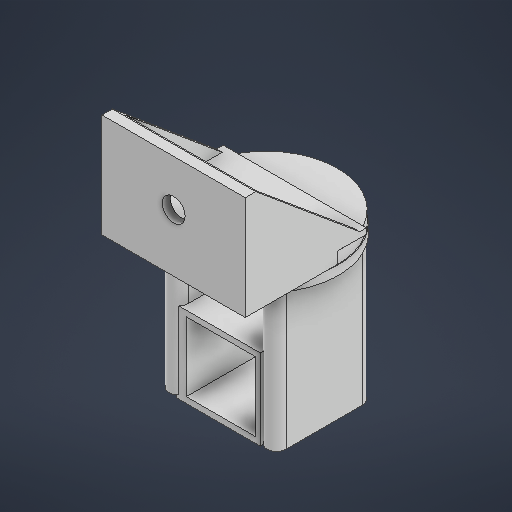
# Autodesk Inventor part: cam_mount0_WITHBASE
Saved by Autodesk Inventor 2027 (Build 310192060, 192F)
## iProperties
Created: 2026-07-16
Part Number: cam_mount0_WITHBASE
Material: Generic
Document SubType Name: Modeling
Designer: farde
Density: 1 g/cm^3
Appearance: Default
Author: farde
Autodesk Inventor part; units mm, degrees
ref_plane "YZ Plane" through (0, 0, 0) normal (1, 0, 0) x (0, 1, 0)
ref_plane "XZ Plane" through (0, 0, 0) normal (0, 1, 0) x (-1, 0, 0)
ref_plane "XY Plane" through (0, 0, 0) normal (0, 0, 1) x (1, 0, 0)
sketch "Sketch1" plane through (0, 0, 0) normal (0, 1, 0) x (-1, 0, 0)
  circle A0 centre (0, 0) radius 25.75
  circle A1 centre (0, 0) radius 23.5
  dimension "d0" = 51.5
  dimension "d1" = 47
  constraints: 2 centre point, 2 coincident
  measures "d0" diameter of A0
  measures "d1" diameter of A1
extrude "Extrusion1" add sketch "Sketch1" along normal blind 1
sketch "Sketch2" plane through (0, 0, 0) normal (0, 1, 0) x (-1, 0, 0)
  circle A0 centre (0, 0) radius 31.4135
  circle A1 centre (0, 0) radius 28.9404
  circle A2 centre (0, 0) radius 31.4135
  circle A3 centre (0, 0) radius 20.0919
  dimension "d6" = 40.1837
  constraints: 4 centre point, 4 coincident, 1 concentric
  measures "d6" diameter of A3
extrude "Extrusion2" add sketch "Sketch2" against normal blind 4 contours A0 | A1 | A3
sketch "Sketch3" plane through (0, -4, 0) normal (0, -1, 0) x (1, 0, 0)
  line L0 (21.2066, 16.5968) -> (21.2066, -16.5968) construction
  line L1 (17.0959, 16.5968) -> (17.0959, -16.5968)
  line L2 (25.3174, -16.5968) -> (25.3174, 16.5968)
  arc A0 (25.3174, 16.5968) -> (17.0959, 16.5968) centre (21.2066, 16.5968) ccw
  arc A1 (17.0959, -16.5968) -> (25.3174, -16.5968) centre (21.2066, -16.5968) ccw
  point P0 (0, 0)
  point P1 (21.2066, 0)
  dimension "d28" = 8.2215
  constraints: 8 end point, 4 point on circle, 4 tangent, 2 centre point, 1 midpoint, 1 parallel, 1 vertical
  measures "d28" distance between parallel lines of L1 L2
extrude "Extrusion3" add sketch "Sketch3" along normal blind 60
mirror "Mirror1" about plane through (0, 0, 0) normal (1, 0, 0) of "Extrusion3"
sketch "Sketch4" plane through (0, 0, 0) normal (0, 1, 0) x (1, 0, 0)
  circle A0 centre (0, 0) radius 17.5
  dimension "d11" = 35
  constraints: 1 centre point, 1 coincident
  measures "d11" diameter of A0
extrude "Extrusion4" cut sketch "Sketch4" against normal blind 60
sketch "Sketch5" plane through (17.0959, -64, -16.5968) normal (-1, 0, 0) x (0, 0, 1)
  line L0 (36.0968, -1.5251) -> (1.0968, -1.5251)
  line L1 (1.0968, -1.5251) -> (1.0968, 33.4749)
  line L2 (1.0968, 33.4749) -> (36.0968, 33.4749)
  line L3 (36.0968, 33.4749) -> (36.0968, -1.5251)
  line L4 (36.0968, -1.5251) -> (1.0968, 33.4749) construction
  line L5 (1.0968, -1.5251) -> (36.0968, 33.4749) construction
  point P0 (16.5968, 64)
  point P1 (18.5968, 15.9749)
  dimension "d12" = 35
  dimension "d13" = 35
  constraints: 12 end point, 2 midpoint, 2 parallel, 1 horizontal, 1 perpendicular
  measures "d12" distance of L1.end L2.end
  measures "d13" distance of L0.end L1.end
extrude "Extrusion5" add sketch "Sketch5" along normal blind 36.1875
sketch "Sketch6" plane through (17.0959, -65.5251, -15.5) normal (0, -1, 0) x (1, 0, 0)
  point P0 (-17.0959, 15.5)
sketch "Sketch8" plane through (-25.3174, -64, -16.5968) normal (-1, 0, 0) x (0, 0, 1)
  line L0 (11.7088, 49.275) -> (100.4099, 49.275) construction
  line L1 (100.4099, 49.275) -> (100.4099, -15.6082) construction
  line L2 (100.4099, -15.6082) -> (11.7088, -15.6082) construction
  line L3 (11.7088, -15.6082) -> (11.7088, 49.275) construction
  spline S0 degree 2 poles (19.8761, 43.1638) (19.8761, 40.0035) (18.0389, 37.0431) (16.1256, 37.0431) knots 0 0 0 1 2 2 2
  spline S1 degree 2 poles (16.1256, 37.0431) (14.1837, 37.0431) (12.3656, 40.0606) (12.3656, 43.1543) knots 0 0 0 1 2 2 2
  spline S2 degree 2 poles (12.3656, 43.1543) (12.3656, 46.3337) (14.2027, 49.275) (16.1256, 49.275) knots 0 0 0 1 2 2 2
  spline S3 degree 2 poles (16.1256, 49.275) (18.0579, 49.275) (19.8761, 46.2289) (19.8761, 43.1638) knots 0 0 0 1 2 2 2
  spline S4 degree 2 poles (17.858, 39.5847) (18.0865, 40.1653) (18.2769, 41.9549) (18.2769, 43.1638) knots 0 0 0 1 2 2 2
  spline S5 degree 2 poles (18.2769, 43.1638) (18.2769, 44.3727) (18.0865, 46.1528) (17.8485, 46.7525) knots 0 0 0 1 2 2 2
  spline S6 degree 2 poles (17.8485, 46.7525) (17.6106, 47.3522) (16.7824, 47.9709) (16.1256, 47.9709) knots 0 0 0 1 2 2 2
  spline S7 degree 2 poles (16.1256, 47.9709) (15.4688, 47.9709) (14.6216, 47.3522) (14.3741, 46.7335) knots 0 0 0 1 2 2 2
  spline S8 degree 2 poles (14.3741, 46.7335) (14.1361, 46.1338) (13.9648, 44.3061) (13.9648, 43.1543) knots 0 0 0 1 2 2 2
  spline S9 degree 2 poles (13.9648, 43.1543) (13.9648, 41.9168) (14.1171, 40.2605) (14.3646, 39.6132) knots 0 0 0 1 2 2 2
  spline S10 degree 2 poles (14.3646, 39.6132) (14.593, 39.004) (15.4402, 38.3472) (16.1256, 38.3472) knots 0 0 0 1 2 2 2
  spline S11 degree 2 poles (16.1256, 38.3472) (16.7729, 38.3472) (17.6201, 38.9659) (17.858, 39.5847) knots 0 0 0 1 2 2 2
  spline S12 degree 2 poles (27.3295, 46.2385) (27.3295, 44.9724) (25.597, 43.24) (24.331, 43.24) knots 0 0 0 1 2 2 2
  spline S13 degree 2 poles (24.331, 43.24) (23.0745, 43.24) (21.323, 44.9629) (21.323, 46.2385) knots 0 0 0 1 2 2 2
  spline S14 degree 2 poles (21.323, 46.2385) (21.323, 47.5045) (23.0554, 49.237) (24.331, 49.237) knots 0 0 0 1 2 2 2
  spline S15 degree 2 poles (24.331, 49.237) (25.597, 49.237) (27.3295, 47.5045) (27.3295, 46.2385) knots 0 0 0 1 2 2 2
  spline S16 degree 2 poles (26.092, 46.2385) (26.092, 47) (25.083, 48.0376) (24.331, 48.0376) knots 0 0 0 1 2 2 2
  spline S17 degree 2 poles (24.331, 48.0376) (23.5695, 48.0376) (22.5604, 47) (22.5604, 46.2385) knots 0 0 0 1 2 2 2
  spline S18 degree 2 poles (22.5604, 46.2385) (22.5604, 45.4674) (23.5885, 44.4394) (24.331, 44.4394) knots 0 0 0 1 2 2 2
  spline S19 degree 2 poles (24.331, 44.4394) (25.083, 44.4394) (26.092, 45.4865) (26.092, 46.2385) knots 0 0 0 1 2 2 2
  point P0 (16.5968, 64)
  constraints: 2 other
sketch "Sketch12" plane through (17.0959, -65.5251, -15.5) normal (0, 0, -1) x (-1, 0, 0)
  line L0 (2.0959, 32.5533) -> (32.0959, 32.5533)
  line L1 (32.0959, 32.5533) -> (32.0959, 2.5533)
  line L2 (32.0959, 2.5533) -> (2.0959, 2.5533)
  line L3 (2.0959, 2.5533) -> (2.0959, 32.5533)
  line L4 (2.0959, 32.5533) -> (32.0959, 2.5533) construction
  line L5 (32.0959, 32.5533) -> (2.0959, 2.5533) construction
  point P0 (17.0959, 65.5251)
  point P1 (17.0959, 17.5533)
  dimension "d35" = 30
  dimension "d36" = 30
  constraints: 12 end point, 2 midpoint, 2 parallel, 1 horizontal, 1 perpendicular
  measures "d35" distance of L1.end L2.end
  measures "d36" distance of L0.end L1.end
extrude "Extrusion10" cut sketch "Sketch12" against normal blind 38.575
sketch "Sketch13" plane through (15, -62.9718, -15.5) normal (-1, 0, 0) x (0, 0, 1)
  line L0 (0, 30) -> (1, 30)
  line L1 (1, 30) -> (1, 27)
  line L2 (1, 27) -> (0, 27)
  line L3 (0, 27) -> (0, 30)
  point P0 (15.5, 62.9718)
  dimension "d39" = 1
  dimension "d40" = 3
  constraints: 8 end point, 2 parallel, 1 horizontal, 1 perpendicular
  measures "d39" distance of L1.end L2.end
  measures "d40" distance of L0.end L1.end
extrude "Extrusion11" add sketch "Sketch13" along normal blind 34.6
sketch "Sketch19" plane through (0, 0, 0) normal (0, 1, 0) x (1, 0, 0)
  arc A0 (31.0588, 0) -> (-31.0588, 0) centre (0, 0) ccw
  line L0 (-31.0588, 0) -> (-31.0588, -40)
  line L1 (31.0588, 0) -> (31.0588, -40)
  line L2 (-31.0588, -40) -> (31.0588, -40)
  dimension "d56" = 40
  dimension "d57" = 40
  constraints: 6 end point, 2 point on circle, 2 vertical, 1 centre point, 1 coincident, 1 perpendicular, 1 tangent
  measures "d56" distance of L0.start L0.end
  measures "d57" distance of L1.start L1.end
extrude "Extrusion17" add sketch "Sketch19" along normal blind 5
sketch "Sketch20" plane through (0, 5, 0) normal (0, 1, 0) x (1, 0, 0)
  line L0 (-31.0588, -40) -> (31.0588, -40) projected
  line L1 (31.0588, -40) -> (-31.0588, -40)
  line L2 (-31.0588, -40) -> (-31.0588, 12.5276)
  line L3 (-31.0588, 12.5276) -> (31.0588, 12.5276)
  line L4 (31.0588, 12.5276) -> (31.0588, -40)
  point P0 (0, 0)
  constraints: 8 end point, 2 parallel, 1 horizontal, 1 perpendicular
extrude "Extrusion18" add sketch "Sketch20" along normal blind 40
sketch "Sketch21" plane through (31.0588, 5, -12.5276) normal (0, 0, -1) x (-1, 0, 0)
  line L0 (2.4864, 37.5821) -> (59.6312, 37.5821)
  line L1 (59.6312, 37.5821) -> (59.6312, 2.4179)
  line L2 (59.6312, 2.4179) -> (2.4864, 2.4179)
  line L3 (2.4864, 2.4179) -> (2.4864, 37.5821)
  line L4 (2.4864, 37.5821) -> (59.6312, 2.4179) construction
  line L5 (59.6312, 37.5821) -> (2.4864, 2.4179) construction
  point P0 (31.0588, -5)
  point P1 (31.0588, 20)
  constraints: 12 end point, 2 midpoint, 2 parallel, 1 horizontal, 1 perpendicular
extrude "Extrusion19" cut sketch "Sketch21" against normal blind 48
sketch "Sketch22" plane through (31.0588, 0, 40) normal (1, 0, 0) x (0, 0, -1)
  line L0 (52.5276, 5) -> (52.5276, 45) projected
  line L1 (4.5275, 45) -> (52.5276, 5)
  line L2 (52.5276, 7.4179) -> (4.5276, 7.4179) projected
  line L3 (52.5276, 45) -> (0, 45) projected
  line L4 (4.5275, 45) -> (52.5276, 45)
  line L5 (71.0588, 5) -> (52.5276, 5) projected
  line L6 (52.5276, 45) -> (52.5276, 5)
  point P0 (40, 0)
  point P1 (4.5275, 45)
  point P2 (49.6261, 7.4179)
  constraints: 6 end point, 1 collinear, 1 perpendicular
extrude "Extrusion20" cut sketch "Sketch22" against normal blind 105.9875 contours L2 L1 L3 L0
sketch "Sketch23" plane through (31.0588, 5, 35.4724) normal (0, 0, -1) x (-1, 0, 0)
  circle A0 centre (31.0588, 20) radius 5
  point P0 (31.0588, -5)
  dimension "d66" = 10
  constraints: 1 centre point
  measures "d66" diameter of A0
extrude "Extrusion21" cut sketch "Sketch23" against normal blind 28.95
sketch "Sketch24" plane through (31.0588, 5, 35.4724) normal (0, 0, -1) x (-1, 0, 0)
  circle A0 centre (31.0588, 20) radius 5 projected
  circle A1 centre (31.0588, 20) radius 9.5
  point P0 (31.0588, -5)
  dimension "d69" = 19
  constraints: 1 centre point, 1 coincident
  measures "d69" diameter of A1
extrude "Extrusion22" cut sketch "Sketch24" against normal blind 1
sketch "Sketch25" plane through (-25.3174, -64, -16.5968) normal (-1, 0, 0) x (0, 0, 1)
  line L0 (7.5258, 35.488) -> (42.1865, 35.488) construction
  line L1 (42.1865, 35.488) -> (42.1865, 27.3803) construction
  line L2 (42.1865, 27.3803) -> (7.5258, 27.3803) construction
  line L3 (7.5258, 27.3803) -> (7.5258, 35.488) construction
  spline S0 degree 2 poles (8.9931, 31.3144) (8.7015, 31.3144) (8.223, 31.4887) (8.0551, 31.6504) knots 0 0 0 1 2 2 2
  spline S1 degree 2 poles (8.0551, 31.6504) (7.8903, 31.8088) (7.7191, 32.2398) (7.7191, 32.4838) knots 0 0 0 1 2 2 2
  spline S2 degree 2 poles (7.7191, 32.4838) (7.7191, 32.8007) (8.0582, 33.3331) (8.3815, 33.4916) knots 0 0 0 1 2 2 2
  line L4 (8.3815, 33.4916) -> (8.3815, 33.5074)
  spline S3 degree 2 poles (8.3815, 33.5074) (8.0931, 33.6754) (7.8142, 34.0747) (7.8142, 34.3725) knots 0 0 0 1 2 2 2
  spline S4 degree 2 poles (7.8142, 34.3725) (7.8142, 34.813) (8.4797, 35.4025) (8.9931, 35.4025) knots 0 0 0 1 2 2 2
  spline S5 degree 2 poles (8.9931, 35.4025) (9.5255, 35.4025) (10.1688, 34.8447) (10.1688, 34.4074) knots 0 0 0 1 2 2 2
  spline S6 degree 2 poles (10.1688, 34.4074) (10.1688, 34.1444) (9.8614, 33.631) (9.573, 33.4852) knots 0 0 0 1 2 2 2
  line L5 (9.573, 33.4852) -> (9.573, 33.4694)
  spline S7 degree 2 poles (9.573, 33.4694) (9.9153, 33.3109) (10.267, 32.8546) (10.267, 32.4933) knots 0 0 0 1 2 2 2
  spline S8 degree 2 poles (10.267, 32.4933) (10.267, 31.9926) (9.5382, 31.3144) (8.9931, 31.3144) knots 0 0 0 1 2 2 2
  spline S9 degree 2 poles (9.7283, 32.4426) (9.7283, 32.6835) (9.5382, 32.9687) (9.2688, 33.1144) knots 0 0 0 1 2 2 2
  spline S10 degree 2 poles (9.2688, 33.1144) (9.1801, 33.1651) (8.8822, 33.2824) (8.6952, 33.3585) knots 0 0 0 1 2 2 2
  spline S11 degree 2 poles (8.6952, 33.3585) (8.4797, 33.2159) (8.2484, 32.7912) (8.2484, 32.5218) knots 0 0 0 1 2 2 2
  spline S12 degree 2 poles (8.2484, 32.5218) (8.2484, 32.1669) (8.6762, 31.7042) (8.9994, 31.7042) knots 0 0 0 1 2 2 2
  spline S13 degree 2 poles (8.9994, 31.7042) (9.329, 31.7042) (9.7283, 32.1004) (9.7283, 32.4426) knots 0 0 0 1 2 2 2
  spline S14 degree 2 poles (9.6554, 34.4011) (9.6554, 34.6641) (9.3036, 35.0159) (8.9899, 35.0159) knots 0 0 0 1 2 2 2
  spline S15 degree 2 poles (8.9899, 35.0159) (8.7047, 35.0159) (8.3403, 34.7021) (8.3403, 34.4328) knots 0 0 0 1 2 2 2
  spline S16 degree 2 poles (8.3403, 34.4328) (8.3403, 34.2394) (8.5272, 33.9701) (8.7142, 33.8623) knots 0 0 0 1 2 2 2
  spline S17 degree 2 poles (8.7142, 33.8623) (8.7934, 33.818) (9.1294, 33.6627) (9.2656, 33.6183) knots 0 0 0 1 2 2 2
  spline S18 degree 2 poles (9.2656, 33.6183) (9.4938, 33.7926) (9.6554, 34.1634) (9.6554, 34.4011) knots 0 0 0 1 2 2 2
  line L6 (12.3713, 35.488) -> (10.8406, 30.5539)
  line L7 (10.8406, 30.5539) -> (10.397, 30.5539)
  line L8 (10.397, 30.5539) -> (11.9213, 35.488)
  line L9 (11.9213, 35.488) -> (12.3713, 35.488)
  line L10 (15.0174, 31.4032) -> (13.1097, 31.4032)
  line L11 (13.1097, 31.4032) -> (13.1097, 31.8025)
  line L12 (13.1097, 31.8025) -> (13.8195, 31.8025)
  line L13 (13.8195, 31.8025) -> (13.8195, 34.4233)
  line L14 (13.8195, 34.4233) -> (13.1097, 34.4233)
  line L15 (13.1097, 34.4233) -> (13.1097, 34.7814)
  spline S19 degree 2 poles (13.1097, 34.7814) (13.5121, 34.7814) (13.8924, 35.0095) (13.9178, 35.3264) knots 0 0 0 1 2 2 2
  line L16 (13.9178, 35.3264) -> (14.3234, 35.3264)
  line L17 (14.3234, 35.3264) -> (14.3234, 31.8025)
  line L18 (14.3234, 31.8025) -> (15.0174, 31.8025)
  line L19 (15.0174, 31.8025) -> (15.0174, 31.4032)
  spline S20 degree 2 poles (16.7921, 34.943) (16.6495, 34.943) (16.3674, 34.8733) (16.2312, 34.8194) knots 0 0 0 1 2 2 2
  spline S21 degree 2 poles (16.2312, 34.8194) (16.1044, 34.7655) (15.9174, 34.6514) (15.8445, 34.6007) knots 0 0 0 1 2 2 2
  line L20 (15.8445, 34.6007) -> (15.8128, 34.6007)
  line L21 (15.8128, 34.6007) -> (15.8128, 35.1553)
  spline S22 degree 2 poles (15.8128, 35.1553) (15.984, 35.2472) (16.5702, 35.3961) (16.8333, 35.3961) knots 0 0 0 1 2 2 2
  spline S23 degree 2 poles (16.8333, 35.3961) (17.0995, 35.3961) (17.4956, 35.2884) (17.6572, 35.1743) knots 0 0 0 1 2 2 2
  spline S24 degree 2 poles (17.6572, 35.1743) (17.8283, 35.0507) (18.0058, 34.6926) (18.0058, 34.4518) knots 0 0 0 1 2 2 2
  spline S25 degree 2 poles (18.0058, 34.4518) (18.0058, 34.1285) (17.5812, 33.6405) (17.2833, 33.5771) knots 0 0 0 1 2 2 2
  line L22 (17.2833, 33.5771) -> (17.2833, 33.5391)
  spline S26 degree 2 poles (17.2833, 33.5391) (17.4069, 33.5137) (17.6889, 33.3997) (17.8093, 33.2856) knots 0 0 0 1 2 2 2
  spline S27 degree 2 poles (17.8093, 33.2856) (17.9298, 33.1747) (18.0819, 32.8197) (18.0819, 32.563) knots 0 0 0 1 2 2 2
  spline S28 degree 2 poles (18.0819, 32.563) (18.0819, 32.3) (17.9012, 31.8532) (17.7364, 31.682) knots 0 0 0 1 2 2 2
  spline S29 degree 2 poles (17.7364, 31.682) (17.5653, 31.5046) (17.0805, 31.3208) (16.7731, 31.3208) knots 0 0 0 1 2 2 2
  spline S30 degree 2 poles (16.7731, 31.3208) (16.4783, 31.3208) (15.9016, 31.4634) (15.7051, 31.5616) knots 0 0 0 1 2 2 2
  line L23 (15.7051, 31.5616) -> (15.7051, 32.1162)
  line L24 (15.7051, 32.1162) -> (15.7431, 32.1162)
  spline S31 degree 2 poles (15.7431, 32.1162) (15.9079, 31.9958) (16.4657, 31.7739) (16.7414, 31.7739) knots 0 0 0 1 2 2 2
  spline S32 degree 2 poles (16.7414, 31.7739) (16.903, 31.7739) (17.2262, 31.8754) (17.334, 31.9926) knots 0 0 0 1 2 2 2
  spline S33 degree 2 poles (17.334, 31.9926) (17.4386, 32.1099) (17.5495, 32.3887) (17.5495, 32.6011) knots 0 0 0 1 2 2 2
  spline S34 degree 2 poles (17.5495, 32.6011) (17.5495, 32.8134) (17.4259, 33.0891) (17.315, 33.1683) knots 0 0 0 1 2 2 2
  spline S35 degree 2 poles (17.315, 33.1683) (17.204, 33.2475) (16.903, 33.3078) (16.7255, 33.3078) knots 0 0 0 1 2 2 2
  line L25 (16.7255, 33.3078) -> (16.5037, 33.3078)
  line L26 (16.5037, 33.3078) -> (16.5037, 33.7419)
  line L27 (16.5037, 33.7419) -> (16.678, 33.7419)
  spline S36 degree 2 poles (16.678, 33.7419) (17.0297, 33.7419) (17.4734, 34.0778) (17.4734, 34.3979) knots 0 0 0 1 2 2 2
  spline S37 degree 2 poles (17.4734, 34.3979) (17.4734, 34.5468) (17.3593, 34.7592) (17.2674, 34.8226) knots 0 0 0 1 2 2 2
  spline S38 degree 2 poles (17.2674, 34.8226) (17.1692, 34.8891) (16.9283, 34.943) (16.7921, 34.943) knots 0 0 0 1 2 2 2
  line L28 (20.297, 35.488) -> (18.7664, 30.5539)
  line L29 (18.7664, 30.5539) -> (18.3227, 30.5539)
  line L30 (18.3227, 30.5539) -> (19.847, 35.488)
  line L31 (19.847, 35.488) -> (20.297, 35.488)
  line L32 (23.1396, 31.4032) -> (20.728, 31.4032)
  line L33 (20.728, 31.4032) -> (20.728, 31.9577)
  spline S39 degree 2 poles (20.728, 31.9577) (20.9879, 32.2018) (21.4505, 32.6549) (21.6724, 32.8989) knots 0 0 0 1 2 2 2
  spline S40 degree 2 poles (21.6724, 32.8989) (22.1192, 33.3901) (22.4456, 33.9796) (22.4456, 34.2933) knots 0 0 0 1 2 2 2
  spline S41 degree 2 poles (22.4456, 34.2933) (22.4456, 34.4581) (22.3442, 34.7053) (22.2523, 34.7845) knots 0 0 0 1 2 2 2
  spline S42 degree 2 poles (22.2523, 34.7845) (22.1604, 34.8637) (21.9196, 34.943) (21.7738, 34.943) knots 0 0 0 1 2 2 2
  spline S43 degree 2 poles (21.7738, 34.943) (21.6343, 34.943) (21.3491, 34.8733) (21.2192, 34.8194) knots 0 0 0 1 2 2 2
  spline S44 degree 2 poles (21.2192, 34.8194) (21.1083, 34.775) (20.9023, 34.6483) (20.8389, 34.6039) knots 0 0 0 1 2 2 2
  line L34 (20.8389, 34.6039) -> (20.8104, 34.6039)
  line L35 (20.8104, 34.6039) -> (20.8104, 35.1616)
  spline S45 degree 2 poles (20.8104, 35.1616) (20.972, 35.2409) (21.552, 35.3961) (21.8118, 35.3961) knots 0 0 0 1 2 2 2
  spline S46 degree 2 poles (21.8118, 35.3961) (22.3601, 35.3961) (22.978, 34.8162) (22.978, 34.3218) knots 0 0 0 1 2 2 2
  spline S47 degree 2 poles (22.978, 34.3218) (22.978, 34.0905) (22.8703, 33.7039) (22.7752, 33.5391) knots 0 0 0 1 2 2 2
  spline S48 degree 2 poles (22.7752, 33.5391) (22.6801, 33.368) (22.4044, 33.032) (22.2523, 32.8704) knots 0 0 0 1 2 2 2
  spline S49 degree 2 poles (22.2523, 32.8704) (22.0051, 32.6011) (21.3998, 32.0243) (21.2192, 31.8563) knots 0 0 0 1 2 2 2
  line L36 (21.2192, 31.8563) -> (23.1396, 31.8563)
  line L37 (23.1396, 31.8563) -> (23.1396, 31.4032)
  spline S50 degree 2 poles (26.1344, 32.6708) (26.1344, 32.3697) (25.9347, 31.8595) (25.7668, 31.6884) knots 0 0 0 1 2 2 2
  spline S51 degree 2 poles (25.7668, 31.6884) (25.5925, 31.5077) (25.1551, 31.3208) (24.8921, 31.3208) knots 0 0 0 1 2 2 2
  spline S52 degree 2 poles (24.8921, 31.3208) (24.6291, 31.3208) (24.1949, 31.4982) (24.0301, 31.6757) knots 0 0 0 1 2 2 2
  spline S53 degree 2 poles (24.0301, 31.6757) (23.8273, 31.888) (23.5991, 32.6011) (23.5991, 33.1208) knots 0 0 0 1 2 2 2
  spline S54 degree 2 poles (23.5991, 33.1208) (23.5991, 33.631) (23.8083, 34.4518) (24.027, 34.756) knots 0 0 0 1 2 2 2
  spline S55 degree 2 poles (24.027, 34.756) (24.2393, 35.0539) (24.9111, 35.3866) (25.3516, 35.3866) knots 0 0 0 1 2 2 2
  spline S56 degree 2 poles (25.3516, 35.3866) (25.4816, 35.3866) (25.7097, 35.3613) (25.7953, 35.3328) knots 0 0 0 1 2 2 2
  line L38 (25.7953, 35.3328) -> (25.7953, 34.8289)
  line L39 (25.7953, 34.8289) -> (25.7731, 34.8289)
  spline S57 degree 2 poles (25.7731, 34.8289) (25.7002, 34.8669) (25.434, 34.9335) (25.2819, 34.9335) knots 0 0 0 1 2 2 2
  spline S58 degree 2 poles (25.2819, 34.9335) (24.7939, 34.9335) (24.1949, 34.2743) (24.1379, 33.6278) knots 0 0 0 1 2 2 2
  spline S59 degree 2 poles (24.1379, 33.6278) (24.3249, 33.7578) (24.7178, 33.9004) (24.9523, 33.9004) knots 0 0 0 1 2 2 2
  spline S60 degree 2 poles (24.9523, 33.9004) (25.1805, 33.9004) (25.5227, 33.8085) (25.7097, 33.669) knots 0 0 0 1 2 2 2
  spline S61 degree 2 poles (25.7097, 33.669) (25.9252, 33.5074) (26.1344, 33.0067) (26.1344, 32.6708) knots 0 0 0 1 2 2 2
  spline S62 degree 2 poles (25.602, 32.6486) (25.602, 32.8894) (25.4752, 33.2159) (25.3358, 33.3299) knots 0 0 0 1 2 2 2
  spline S63 degree 2 poles (25.3358, 33.3299) (25.2312, 33.4123) (24.9713, 33.4662) (24.8351, 33.4662) knots 0 0 0 1 2 2 2
  spline S64 degree 2 poles (24.8351, 33.4662) (24.6513, 33.4662) (24.3058, 33.3553) (24.1379, 33.2507) knots 0 0 0 1 2 2 2
  spline S65 degree 2 poles (24.1379, 33.2507) (24.1347, 33.1937) (24.1284, 33.0859) (24.1284, 33.0035) knots 0 0 0 1 2 2 2
  spline S66 degree 2 poles (24.1284, 33.0035) (24.1284, 32.5979) (24.2868, 32.1004) (24.4073, 31.9704) knots 0 0 0 1 2 2 2
  spline S67 degree 2 poles (24.4073, 31.9704) (24.5182, 31.8468) (24.759, 31.7486) (24.8953, 31.7486) knots 0 0 0 1 2 2 2
  spline S68 degree 2 poles (24.8953, 31.7486) (25.2122, 31.7486) (25.602, 32.1986) (25.602, 32.6486) knots 0 0 0 1 2 2 2
  point P0 (16.5968, 64)
  constraints: 2 other
emboss "Emboss4" sketch "Sketch8" operation add depth 1 direction (1, 0, 0)
emboss "Emboss5" sketch "Sketch25" operation add depth 1 direction (1, 0, 0)
body "Solid1"
